Autodesk Inventor part; units mm, degrees
(part 2 of 2)
sketch "Sketch5" plane through (0, 0, 2) normal (0, 0, 1) x (1, 0, 0)
  line L0 (31.2247, -413) -> (28.338, -408) projected
  line L1 (28.338, -408) -> (31.2247, -403) projected
  line L2 (31.2247, -403) -> (36.9983, -403) projected
  line L3 (36.9983, -403) -> (39.885, -408) projected
  line L4 (39.885, -408) -> (36.9983, -413) projected
  line L5 (36.9983, -413) -> (31.2247, -413) projected
  line L6 (49.9886, -440.5) -> (52.8754, -445.5) projected
  line L7 (52.8754, -445.5) -> (49.9886, -450.5) projected
  line L8 (49.9886, -450.5) -> (44.2151, -450.5) projected
  line L9 (44.2151, -450.5) -> (41.3284, -445.5) projected
  line L10 (41.3284, -445.5) -> (44.2151, -440.5) projected
  line L11 (44.2151, -440.5) -> (49.9886, -440.5) projected
  line L12 (57.2247, -418) -> (62.9983, -418) projected
  line L13 (62.9983, -418) -> (65.885, -423) projected
  line L14 (65.885, -423) -> (62.9983, -428) projected
  line L15 (62.9983, -428) -> (57.2247, -428) projected
  line L16 (57.2247, -428) -> (54.338, -423) projected
  line L17 (54.338, -423) -> (57.2247, -418) projected
  line L18 (78.8754, -430.5) -> (75.9886, -435.5) projected
  line L19 (75.9886, -435.5) -> (70.2151, -435.5) projected
  line L20 (70.2151, -435.5) -> (67.3284, -430.5) projected
  line L21 (67.3284, -430.5) -> (70.2151, -425.5) projected
  line L22 (70.2151, -425.5) -> (75.9886, -425.5) projected
  line L23 (75.9886, -425.5) -> (78.8754, -430.5) projected
  line L24 (80.338, -438) -> (83.2247, -433) projected
  line L25 (83.2247, -433) -> (88.9983, -433) projected
  line L26 (88.9983, -433) -> (91.885, -438) projected
  line L27 (91.885, -438) -> (88.9983, -443) projected
  line L28 (88.9983, -443) -> (83.2247, -443) projected
  line L29 (83.2247, -443) -> (80.338, -438) projected
  line L30 (101.9886, -410.5) -> (104.8754, -415.5) projected
  line L31 (104.8754, -415.5) -> (101.9886, -420.5) projected
  line L32 (101.9886, -420.5) -> (96.2151, -420.5) projected
  line L33 (96.2151, -420.5) -> (93.3284, -415.5) projected
  line L34 (93.3284, -415.5) -> (96.2151, -410.5) projected
  line L35 (96.2151, -410.5) -> (101.9886, -410.5) projected
  line L36 (109.2247, -448) -> (114.9983, -448) projected
  line L37 (114.9983, -448) -> (117.885, -453) projected
  line L38 (117.885, -453) -> (114.9983, -458) projected
  line L39 (114.9983, -458) -> (109.2247, -458) projected
  line L40 (109.2247, -458) -> (106.338, -453) projected
  line L41 (106.338, -453) -> (109.2247, -448) projected
  line L42 (135.2247, -413) -> (132.338, -408) projected
  line L43 (132.338, -408) -> (135.2247, -403) projected
  line L44 (135.2247, -403) -> (140.9983, -403) projected
  line L45 (140.9983, -403) -> (143.885, -408) projected
  line L46 (143.885, -408) -> (140.9983, -413) projected
  line L47 (140.9983, -413) -> (135.2247, -413) projected
  line L48 (153.9886, -440.5) -> (156.8754, -445.5) projected
  line L49 (156.8754, -445.5) -> (153.9886, -450.5) projected
  line L50 (153.9886, -450.5) -> (148.2151, -450.5) projected
  line L51 (148.2151, -450.5) -> (145.3284, -445.5) projected
  line L52 (145.3284, -445.5) -> (148.2151, -440.5) projected
  line L53 (148.2151, -440.5) -> (153.9886, -440.5) projected
  line L54 (153.9886, -410.5) -> (156.8754, -415.5) projected
  line L55 (156.8754, -415.5) -> (153.9886, -420.5) projected
  line L56 (153.9886, -420.5) -> (148.2151, -420.5) projected
  line L57 (148.2151, -420.5) -> (145.3284, -415.5) projected
  line L58 (145.3284, -415.5) -> (148.2151, -410.5) projected
  line L59 (148.2151, -410.5) -> (153.9886, -410.5) projected
  line L60 (182.8754, -430.5) -> (179.9886, -435.5) projected
  line L61 (179.9886, -435.5) -> (174.2151, -435.5) projected
  line L62 (174.2151, -435.5) -> (171.3284, -430.5) projected
  line L63 (171.3284, -430.5) -> (174.2151, -425.5) projected
  line L64 (174.2151, -425.5) -> (179.9886, -425.5) projected
  line L65 (179.9886, -425.5) -> (182.8754, -430.5) projected
  line L66 (184.338, -438) -> (187.2247, -433) projected
  line L67 (187.2247, -433) -> (192.9983, -433) projected
  line L68 (192.9983, -433) -> (195.885, -438) projected
  line L69 (195.885, -438) -> (192.9983, -443) projected
  line L70 (192.9983, -443) -> (187.2247, -443) projected
  line L71 (187.2247, -443) -> (184.338, -438) projected
  line L72 (205.9886, -410.5) -> (208.8754, -415.5) projected
  line L73 (208.8754, -415.5) -> (205.9886, -420.5) projected
  line L74 (205.9886, -420.5) -> (200.2151, -420.5) projected
  line L75 (200.2151, -420.5) -> (197.3284, -415.5) projected
  line L76 (197.3284, -415.5) -> (200.2151, -410.5) projected
  line L77 (200.2151, -410.5) -> (205.9886, -410.5) projected
  line L78 (213.2247, -448) -> (218.9983, -448) projected
  line L79 (218.9983, -448) -> (221.885, -453) projected
  line L80 (221.885, -453) -> (218.9983, -458) projected
  line L81 (218.9983, -458) -> (213.2247, -458) projected
  line L82 (213.2247, -458) -> (210.338, -453) projected
  line L83 (210.338, -453) -> (213.2247, -448) projected
  line L84 (239.2247, -413) -> (236.338, -408) projected
  line L85 (236.338, -408) -> (239.2247, -403) projected
  line L86 (239.2247, -403) -> (244.9983, -403) projected
  line L87 (244.9983, -403) -> (247.885, -408) projected
  line L88 (247.885, -408) -> (244.9983, -413) projected
  line L89 (244.9983, -413) -> (239.2247, -413) projected
  line L90 (257.9886, -440.5) -> (260.8754, -445.5) projected
  line L91 (260.8754, -445.5) -> (257.9886, -450.5) projected
  line L92 (257.9886, -450.5) -> (252.2151, -450.5) projected
  line L93 (252.2151, -450.5) -> (249.3284, -445.5) projected
  line L94 (249.3284, -445.5) -> (252.2151, -440.5) projected
  line L95 (252.2151, -440.5) -> (257.9886, -440.5) projected
  line L96 (265.2247, -418) -> (270.9983, -418) projected
  line L97 (270.9983, -418) -> (273.885, -423) projected
  line L98 (273.885, -423) -> (270.9983, -428) projected
  line L99 (270.9983, -428) -> (265.2247, -428) projected
  line L100 (265.2247, -428) -> (262.338, -423) projected
  line L101 (262.338, -423) -> (265.2247, -418) projected
  line L102 (291.2247, -448) -> (296.9983, -448) projected
  line L103 (296.9983, -448) -> (299.885, -453) projected
  line L104 (299.885, -453) -> (296.9983, -458) projected
  line L105 (296.9983, -458) -> (291.2247, -458) projected
  line L106 (291.2247, -458) -> (288.338, -453) projected
  line L107 (288.338, -453) -> (291.2247, -448) projected
  line L108 (343.2247, -448) -> (348.9983, -448) projected
  line L109 (348.9983, -448) -> (351.885, -453) projected
  line L110 (351.885, -453) -> (348.9983, -458) projected
  line L111 (348.9983, -458) -> (343.2247, -458) projected
  line L112 (343.2247, -458) -> (340.338, -453) projected
  line L113 (340.338, -453) -> (343.2247, -448) projected
  line L114 (335.9886, -410.5) -> (338.8754, -415.5) projected
  line L115 (338.8754, -415.5) -> (335.9886, -420.5) projected
  line L116 (335.9886, -420.5) -> (330.2151, -420.5) projected
  line L117 (330.2151, -420.5) -> (327.3284, -415.5) projected
  line L118 (327.3284, -415.5) -> (330.2151, -410.5) projected
  line L119 (330.2151, -410.5) -> (335.9886, -410.5) projected
  line L120 (286.8754, -430.5) -> (283.9886, -435.5) projected
  line L121 (283.9886, -435.5) -> (278.2151, -435.5) projected
  line L122 (278.2151, -435.5) -> (275.3284, -430.5) projected
  line L123 (275.3284, -430.5) -> (278.2151, -425.5) projected
  line L124 (278.2151, -425.5) -> (283.9886, -425.5) projected
  line L125 (283.9886, -425.5) -> (286.8754, -430.5) projected
  line L126 (309.9886, -410.5) -> (312.8754, -415.5) projected
  line L127 (312.8754, -415.5) -> (309.9886, -420.5) projected
  line L128 (309.9886, -420.5) -> (304.2151, -420.5) projected
  line L129 (304.2151, -420.5) -> (301.3284, -415.5) projected
  line L130 (301.3284, -415.5) -> (304.2151, -410.5) projected
  line L131 (304.2151, -410.5) -> (309.9886, -410.5) projected
  line L132 (5.2247, -433) -> (10.9983, -433) projected
  line L133 (10.9983, -433) -> (13.885, -438) projected
  line L134 (13.885, -438) -> (10.9983, -443) projected
  line L135 (10.9983, -443) -> (5.2247, -443) projected
  line L136 (5.2247, -443) -> (2.338, -438) projected
  line L137 (2.338, -438) -> (5.2247, -433) projected
  line L138 (23.9886, -440.5) -> (26.8754, -445.5) projected
  line L139 (26.8754, -445.5) -> (23.9886, -450.5) projected
  line L140 (23.9886, -450.5) -> (18.2151, -450.5) projected
  line L141 (18.2151, -450.5) -> (15.3284, -445.5) projected
  line L142 (15.3284, -445.5) -> (18.2151, -440.5) projected
  line L143 (18.2151, -440.5) -> (23.9886, -440.5) projected
  line L144 (10.9983, -428) -> (5.2247, -428) projected
  line L145 (5.2247, -428) -> (2.338, -423) projected
  line L146 (2.338, -423) -> (5.2247, -418) projected
  line L147 (5.2247, -418) -> (10.9983, -418) projected
  line L148 (10.9983, -418) -> (13.885, -423) projected
  line L149 (13.885, -423) -> (10.9983, -428) projected
  line L150 (317.2247, -418) -> (322.9983, -418) projected
  line L151 (322.9983, -418) -> (325.885, -423) projected
  line L152 (325.885, -423) -> (322.9983, -428) projected
  line L153 (322.9983, -428) -> (317.2247, -428) projected
  line L154 (317.2247, -428) -> (314.338, -423) projected
  line L155 (314.338, -423) -> (317.2247, -418) projected
  line L156 (291.2247, -418) -> (296.9983, -418) projected
  line L157 (296.9983, -418) -> (299.885, -423) projected
  line L158 (299.885, -423) -> (296.9983, -428) projected
  line L159 (296.9983, -428) -> (291.2247, -428) projected
  line L160 (291.2247, -428) -> (288.338, -423) projected
  line L161 (288.338, -423) -> (291.2247, -418) projected
  line L162 (317.2247, -413) -> (314.338, -408) projected
  line L163 (314.338, -408) -> (317.2247, -403) projected
  line L164 (317.2247, -403) -> (322.9983, -403) projected
  line L165 (322.9983, -403) -> (325.885, -408) projected
  line L166 (325.885, -408) -> (322.9983, -413) projected
  line L167 (322.9983, -413) -> (317.2247, -413) projected
  line L168 (340.338, -438) -> (343.2247, -433) projected
  line L169 (343.2247, -433) -> (348.9983, -433) projected
  line L170 (348.9983, -433) -> (351.885, -438) projected
  line L171 (351.885, -438) -> (348.9983, -443) projected
  line L172 (348.9983, -443) -> (343.2247, -443) projected
  line L173 (343.2247, -443) -> (340.338, -438) projected
  line L174 (309.9886, -440.5) -> (312.8754, -445.5) projected
  line L175 (312.8754, -445.5) -> (309.9886, -450.5) projected
  line L176 (309.9886, -450.5) -> (304.2151, -450.5) projected
  line L177 (304.2151, -450.5) -> (301.3284, -445.5) projected
  line L178 (301.3284, -445.5) -> (304.2151, -440.5) projected
  line L179 (304.2151, -440.5) -> (309.9886, -440.5) projected
  line L180 (262.338, -438) -> (265.2247, -433) projected
  line L181 (265.2247, -433) -> (270.9983, -433) projected
  line L182 (270.9983, -433) -> (273.885, -438) projected
  line L183 (273.885, -438) -> (270.9983, -443) projected
  line L184 (270.9983, -443) -> (265.2247, -443) projected
  line L185 (265.2247, -443) -> (262.338, -438) projected
  line L186 (260.8754, -430.5) -> (257.9886, -435.5) projected
  line L187 (257.9886, -435.5) -> (252.2151, -435.5) projected
  line L188 (252.2151, -435.5) -> (249.3284, -430.5) projected
  line L189 (249.3284, -430.5) -> (252.2151, -425.5) projected
  line L190 (252.2151, -425.5) -> (257.9886, -425.5) projected
  line L191 (257.9886, -425.5) -> (260.8754, -430.5) projected
  line L192 (239.2247, -418) -> (244.9983, -418) projected
  line L193 (244.9983, -418) -> (247.885, -423) projected
  line L194 (247.885, -423) -> (244.9983, -428) projected
  line L195 (244.9983, -428) -> (239.2247, -428) projected
  line L196 (239.2247, -428) -> (236.338, -423) projected
  line L197 (236.338, -423) -> (239.2247, -418) projected
  line L198 (231.9886, -440.5) -> (234.8754, -445.5) projected
  line L199 (234.8754, -445.5) -> (231.9886, -450.5) projected
  line L200 (231.9886, -450.5) -> (226.2151, -450.5) projected
  line L201 (226.2151, -450.5) -> (223.3284, -445.5) projected
  line L202 (223.3284, -445.5) -> (226.2151, -440.5) projected
  line L203 (226.2151, -440.5) -> (231.9886, -440.5) projected
  line L204 (213.2247, -413) -> (210.338, -408) projected
  line L205 (210.338, -408) -> (213.2247, -403) projected
  line L206 (213.2247, -403) -> (218.9983, -403) projected
  line L207 (218.9983, -403) -> (221.885, -408) projected
  line L208 (221.885, -408) -> (218.9983, -413) projected
  line L209 (218.9983, -413) -> (213.2247, -413) projected
  line L210 (187.2247, -448) -> (192.9983, -448) projected
  line L211 (192.9983, -448) -> (195.885, -453) projected
  line L212 (195.885, -453) -> (192.9983, -458) projected
  line L213 (192.9983, -458) -> (187.2247, -458) projected
  line L214 (187.2247, -458) -> (184.338, -453) projected
  line L215 (184.338, -453) -> (187.2247, -448) projected
  line L216 (179.9886, -410.5) -> (182.8754, -415.5) projected
  line L217 (182.8754, -415.5) -> (179.9886, -420.5) projected
  line L218 (179.9886, -420.5) -> (174.2151, -420.5) projected
  line L219 (174.2151, -420.5) -> (171.3284, -415.5) projected
  line L220 (171.3284, -415.5) -> (174.2151, -410.5) projected
  line L221 (174.2151, -410.5) -> (179.9886, -410.5) projected
  line L222 (161.2247, -413) -> (158.338, -408) projected
  line L223 (158.338, -408) -> (161.2247, -403) projected
  line L224 (161.2247, -403) -> (166.9983, -403) projected
  line L225 (166.9983, -403) -> (169.885, -408) projected
  line L226 (169.885, -408) -> (166.9983, -413) projected
  line L227 (166.9983, -413) -> (161.2247, -413) projected
  line L228 (161.2247, -448) -> (166.9983, -448) projected
  line L229 (166.9983, -448) -> (169.885, -453) projected
  line L230 (169.885, -453) -> (166.9983, -458) projected
  line L231 (166.9983, -458) -> (161.2247, -458) projected
  line L232 (161.2247, -458) -> (158.338, -453) projected
  line L233 (158.338, -453) -> (161.2247, -448) projected
  line L234 (135.2247, -418) -> (140.9983, -418) projected
  line L235 (140.9983, -418) -> (143.885, -423) projected
  line L236 (143.885, -423) -> (140.9983, -428) projected
  line L237 (140.9983, -428) -> (135.2247, -428) projected
  line L238 (135.2247, -428) -> (132.338, -423) projected
  line L239 (132.338, -423) -> (135.2247, -418) projected
  line L240 (127.9886, -440.5) -> (130.8754, -445.5) projected
  line L241 (130.8754, -445.5) -> (127.9886, -450.5) projected
  line L242 (127.9886, -450.5) -> (122.2151, -450.5) projected
  line L243 (122.2151, -450.5) -> (119.3284, -445.5) projected
  line L244 (119.3284, -445.5) -> (122.2151, -440.5) projected
  line L245 (122.2151, -440.5) -> (127.9886, -440.5) projected
  line L246 (109.2247, -413) -> (106.338, -408) projected
  line L247 (106.338, -408) -> (109.2247, -403) projected
  line L248 (109.2247, -403) -> (114.9983, -403) projected
  line L249 (114.9983, -403) -> (117.885, -408) projected
  line L250 (117.885, -408) -> (114.9983, -413) projected
  line L251 (114.9983, -413) -> (109.2247, -413) projected
  line L252 (83.2247, -448) -> (88.9983, -448) projected
  line L253 (88.9983, -448) -> (91.885, -453) projected
  line L254 (91.885, -453) -> (88.9983, -458) projected
  line L255 (88.9983, -458) -> (83.2247, -458) projected
  line L256 (83.2247, -458) -> (80.338, -453) projected
  line L257 (80.338, -453) -> (83.2247, -448) projected
  line L258 (75.9886, -410.5) -> (78.8754, -415.5) projected
  line L259 (78.8754, -415.5) -> (75.9886, -420.5) projected
  line L260 (75.9886, -420.5) -> (70.2151, -420.5) projected
  line L261 (70.2151, -420.5) -> (67.3284, -415.5) projected
  line L262 (67.3284, -415.5) -> (70.2151, -410.5) projected
  line L263 (70.2151, -410.5) -> (75.9886, -410.5) projected
  line L264 (54.338, -438) -> (57.2247, -433) projected
  line L265 (57.2247, -433) -> (62.9983, -433) projected
  line L266 (62.9983, -433) -> (65.885, -438) projected
  line L267 (65.885, -438) -> (62.9983, -443) projected
  line L268 (62.9983, -443) -> (57.2247, -443) projected
  line L269 (57.2247, -443) -> (54.338, -438) projected
  line L270 (52.8754, -430.5) -> (49.9886, -435.5) projected
  line L271 (49.9886, -435.5) -> (44.2151, -435.5) projected
  line L272 (44.2151, -435.5) -> (41.3284, -430.5) projected
  line L273 (41.3284, -430.5) -> (44.2151, -425.5) projected
  line L274 (44.2151, -425.5) -> (49.9886, -425.5) projected
  line L275 (49.9886, -425.5) -> (52.8754, -430.5) projected
  line L276 (31.2247, -418) -> (36.9983, -418) projected
  line L277 (36.9983, -418) -> (39.885, -423) projected
  line L278 (39.885, -423) -> (36.9983, -428) projected
  line L279 (36.9983, -428) -> (31.2247, -428) projected
  line L280 (31.2247, -428) -> (28.338, -423) projected
  line L281 (28.338, -423) -> (31.2247, -418) projected
  line L282 (23.9886, -420.5) -> (18.2151, -420.5) projected
  line L283 (18.2151, -420.5) -> (15.3284, -415.5) projected
  line L284 (15.3284, -415.5) -> (18.2151, -410.5) projected
  line L285 (18.2151, -410.5) -> (23.9886, -410.5) projected
  line L286 (23.9886, -410.5) -> (26.8754, -415.5) projected
  line L287 (26.8754, -415.5) -> (23.9886, -420.5) projected
  line L288 (31.2247, -448) -> (36.9983, -448) projected
  line L289 (36.9983, -448) -> (39.885, -453) projected
  line L290 (39.885, -453) -> (36.9983, -458) projected
  line L291 (36.9983, -458) -> (31.2247, -458) projected
  line L292 (31.2247, -458) -> (28.338, -453) projected
  line L293 (28.338, -453) -> (31.2247, -448) projected
  line L294 (57.2247, -413) -> (54.338, -408) projected
  line L295 (54.338, -408) -> (57.2247, -403) projected
  line L296 (57.2247, -403) -> (62.9983, -403) projected
  line L297 (62.9983, -403) -> (65.885, -408) projected
  line L298 (65.885, -408) -> (62.9983, -413) projected
  line L299 (62.9983, -413) -> (57.2247, -413) projected
  line L300 (75.9886, -440.5) -> (78.8754, -445.5) projected
  line L301 (78.8754, -445.5) -> (75.9886, -450.5) projected
  line L302 (75.9886, -450.5) -> (70.2151, -450.5) projected
  line L303 (70.2151, -450.5) -> (67.3284, -445.5) projected
  line L304 (67.3284, -445.5) -> (70.2151, -440.5) projected
  line L305 (70.2151, -440.5) -> (75.9886, -440.5) projected
  line L306 (83.2247, -418) -> (88.9983, -418) projected
  line L307 (88.9983, -418) -> (91.885, -423) projected
  line L308 (91.885, -423) -> (88.9983, -428) projected
  line L309 (88.9983, -428) -> (83.2247, -428) projected
  line L310 (83.2247, -428) -> (80.338, -423) projected
  line L311 (80.338, -423) -> (83.2247, -418) projected
  line L312 (104.8754, -430.5) -> (101.9886, -435.5) projected
  line L313 (101.9886, -435.5) -> (96.2151, -435.5) projected
  line L314 (96.2151, -435.5) -> (93.3284, -430.5) projected
  line L315 (93.3284, -430.5) -> (96.2151, -425.5) projected
  line L316 (96.2151, -425.5) -> (101.9886, -425.5) projected
  line L317 (101.9886, -425.5) -> (104.8754, -430.5) projected
  line L318 (106.338, -438) -> (109.2247, -433) projected
  line L319 (109.2247, -433) -> (114.9983, -433) projected
  line L320 (114.9983, -433) -> (117.885, -438) projected
  line L321 (117.885, -438) -> (114.9983, -443) projected
  line L322 (114.9983, -443) -> (109.2247, -443) projected
  line L323 (109.2247, -443) -> (106.338, -438) projected
  line L324 (127.9886, -410.5) -> (130.8754, -415.5) projected
  line L325 (130.8754, -415.5) -> (127.9886, -420.5) projected
  line L326 (127.9886, -420.5) -> (122.2151, -420.5) projected
  line L327 (122.2151, -420.5) -> (119.3284, -415.5) projected
  line L328 (119.3284, -415.5) -> (122.2151, -410.5) projected
  line L329 (122.2151, -410.5) -> (127.9886, -410.5) projected
  line L330 (135.2247, -448) -> (140.9983, -448) projected
  line L331 (140.9983, -448) -> (143.885, -453) projected
  line L332 (143.885, -453) -> (140.9983, -458) projected
  line L333 (140.9983, -458) -> (135.2247, -458) projected
  line L334 (135.2247, -458) -> (132.338, -453) projected
  line L335 (132.338, -453) -> (135.2247, -448) projected
  line L336 (156.8754, -430.5) -> (153.9886, -435.5) projected
  line L337 (153.9886, -435.5) -> (148.2151, -435.5) projected
  line L338 (148.2151, -435.5) -> (145.3284, -430.5) projected
  line L339 (145.3284, -430.5) -> (148.2151, -425.5) projected
  line L340 (148.2151, -425.5) -> (153.9886, -425.5) projected
  line L341 (153.9886, -425.5) -> (156.8754, -430.5) projected
  line L342 (179.9886, -440.5) -> (182.8754, -445.5) projected
  line L343 (182.8754, -445.5) -> (179.9886, -450.5) projected
  line L344 (179.9886, -450.5) -> (174.2151, -450.5) projected
  line L345 (174.2151, -450.5) -> (171.3284, -445.5) projected
  line L346 (171.3284, -445.5) -> (174.2151, -440.5) projected
  line L347 (174.2151, -440.5) -> (179.9886, -440.5) projected
  line L348 (187.2247, -418) -> (192.9983, -418) projected
  line L349 (192.9983, -418) -> (195.885, -423) projected
  line L350 (195.885, -423) -> (192.9983, -428) projected
  line L351 (192.9983, -428) -> (187.2247, -428) projected
  line L352 (187.2247, -428) -> (184.338, -423) projected
  line L353 (184.338, -423) -> (187.2247, -418) projected
  line L354 (208.8754, -430.5) -> (205.9886, -435.5) projected
  line L355 (205.9886, -435.5) -> (200.2151, -435.5) projected
  line L356 (200.2151, -435.5) -> (197.3284, -430.5) projected
  line L357 (197.3284, -430.5) -> (200.2151, -425.5) projected
  line L358 (200.2151, -425.5) -> (205.9886, -425.5) projected
  line L359 (205.9886, -425.5) -> (208.8754, -430.5) projected
  line L360 (210.338, -438) -> (213.2247, -433) projected
  line L361 (213.2247, -433) -> (218.9983, -433) projected
  line L362 (218.9983, -433) -> (221.885, -438) projected
  line L363 (221.885, -438) -> (218.9983, -443) projected
  line L364 (218.9983, -443) -> (213.2247, -443) projected
  line L365 (213.2247, -443) -> (210.338, -438) projected
  line L366 (231.9886, -410.5) -> (234.8754, -415.5) projected
  line L367 (234.8754, -415.5) -> (231.9886, -420.5) projected
  line L368 (231.9886, -420.5) -> (226.2151, -420.5) projected
  line L369 (226.2151, -420.5) -> (223.3284, -415.5) projected
  line L370 (223.3284, -415.5) -> (226.2151, -410.5) projected
  line L371 (226.2151, -410.5) -> (231.9886, -410.5) projected
  line L372 (239.2247, -448) -> (244.9983, -448) projected
  line L373 (244.9983, -448) -> (247.885, -453) projected
  line L374 (247.885, -453) -> (244.9983, -458) projected
  line L375 (244.9983, -458) -> (239.2247, -458) projected
  line L376 (239.2247, -458) -> (236.338, -453) projected
  line L377 (236.338, -453) -> (239.2247, -448) projected
  line L378 (265.2247, -413) -> (262.338, -408) projected
  line L379 (262.338, -408) -> (265.2247, -403) projected
  line L380 (265.2247, -403) -> (270.9983, -403) projected
  line L381 (270.9983, -403) -> (273.885, -408) projected
  line L382 (273.885, -408) -> (270.9983, -413) projected
  line L383 (270.9983, -413) -> (265.2247, -413) projected
  line L384 (283.9886, -440.5) -> (286.8754, -445.5) projected
  line L385 (286.8754, -445.5) -> (283.9886, -450.5) projected
  line L386 (283.9886, -450.5) -> (278.2151, -450.5) projected
  line L387 (278.2151, -450.5) -> (275.3284, -445.5) projected
  line L388 (275.3284, -445.5) -> (278.2151, -440.5) projected
  line L389 (278.2151, -440.5) -> (283.9886, -440.5) projected
  line L390 (335.9886, -440.5) -> (338.8754, -445.5) projected
  line L391 (338.8754, -445.5) -> (335.9886, -450.5) projected
  line L392 (335.9886, -450.5) -> (330.2151, -450.5) projected
  line L393 (330.2151, -450.5) -> (327.3284, -445.5) projected
  line L394 (327.3284, -445.5) -> (330.2151, -440.5) projected
  line L395 (330.2151, -440.5) -> (335.9886, -440.5) projected
  line L396 (343.2247, -413) -> (340.338, -408) projected
  line L397 (340.338, -408) -> (343.2247, -403) projected
  line L398 (343.2247, -403) -> (348.9983, -403) projected
  line L399 (348.9983, -403) -> (351.885, -408) projected
  line L400 (351.885, -408) -> (348.9983, -413) projected
  line L401 (348.9983, -413) -> (343.2247, -413) projected
  line L402 (283.9886, -410.5) -> (286.8754, -415.5) projected
  line L403 (286.8754, -415.5) -> (283.9886, -420.5) projected
  line L404 (283.9886, -420.5) -> (278.2151, -420.5) projected
  line L405 (278.2151, -420.5) -> (275.3284, -415.5) projected
  line L406 (275.3284, -415.5) -> (278.2151, -410.5) projected
  line L407 (278.2151, -410.5) -> (283.9886, -410.5) projected
  line L408 (312.8754, -430.5) -> (309.9886, -435.5) projected
  line L409 (309.9886, -435.5) -> (304.2151, -435.5) projected
  line L410 (304.2151, -435.5) -> (301.3284, -430.5) projected
  line L411 (301.3284, -430.5) -> (304.2151, -425.5) projected
  line L412 (304.2151, -425.5) -> (309.9886, -425.5) projected
  line L413 (309.9886, -425.5) -> (312.8754, -430.5) projected
  line L414 (338.8754, -430.5) -> (335.9886, -435.5) projected
  line L415 (335.9886, -435.5) -> (330.2151, -435.5) projected
  line L416 (330.2151, -435.5) -> (327.3284, -430.5) projected
  line L417 (327.3284, -430.5) -> (330.2151, -425.5) projected
  line L418 (330.2151, -425.5) -> (335.9886, -425.5) projected
  line L419 (335.9886, -425.5) -> (338.8754, -430.5) projected
  line L420 (23.9886, -435.5) -> (18.2151, -435.5) projected
  line L421 (18.2151, -435.5) -> (15.3284, -430.5) projected
  line L422 (15.3284, -430.5) -> (18.2151, -425.5) projected
  line L423 (18.2151, -425.5) -> (23.9886, -425.5) projected
  line L424 (23.9886, -425.5) -> (26.8754, -430.5) projected
  line L425 (26.8754, -430.5) -> (23.9886, -435.5) projected
  line L426 (5.2247, -448) -> (10.9983, -448) projected
  line L427 (10.9983, -448) -> (13.885, -453) projected
  line L428 (13.885, -453) -> (10.9983, -458) projected
  line L429 (10.9983, -458) -> (5.2247, -458) projected
  line L430 (5.2247, -458) -> (2.338, -453) projected
  line L431 (2.338, -453) -> (5.2247, -448) projected
  line L432 (314.338, -438) -> (317.2247, -433) projected
  line L433 (317.2247, -433) -> (322.9983, -433) projected
  line L434 (322.9983, -433) -> (325.885, -438) projected
  line L435 (325.885, -438) -> (322.9983, -443) projected
  line L436 (322.9983, -443) -> (317.2247, -443) projected
  line L437 (317.2247, -443) -> (314.338, -438) projected
  line L438 (288.338, -438) -> (291.2247, -433) projected
  line L439 (291.2247, -433) -> (296.9983, -433) projected
  line L440 (296.9983, -433) -> (299.885, -438) projected
  line L441 (299.885, -438) -> (296.9983, -443) projected
  line L442 (296.9983, -443) -> (291.2247, -443) projected
  line L443 (291.2247, -443) -> (288.338, -438) projected
  line L444 (291.2247, -413) -> (288.338, -408) projected
  line L445 (288.338, -408) -> (291.2247, -403) projected
  line L446 (291.2247, -403) -> (296.9983, -403) projected
  line L447 (296.9983, -403) -> (299.885, -408) projected
  line L448 (299.885, -408) -> (296.9983, -413) projected
  line L449 (296.9983, -413) -> (291.2247, -413) projected
  line L450 (343.2247, -418) -> (348.9983, -418) projected
  line L451 (348.9983, -418) -> (351.885, -423) projected
  line L452 (351.885, -423) -> (348.9983, -428) projected
  line L453 (348.9983, -428) -> (343.2247, -428) projected
  line L454 (343.2247, -428) -> (340.338, -423) projected
  line L455 (340.338, -423) -> (343.2247, -418) projected
  line L456 (317.2247, -448) -> (322.9983, -448) projected
  line L457 (322.9983, -448) -> (325.885, -453) projected
  line L458 (325.885, -453) -> (322.9983, -458) projected
  line L459 (322.9983, -458) -> (317.2247, -458) projected
  line L460 (317.2247, -458) -> (314.338, -453) projected
  line L461 (314.338, -453) -> (317.2247, -448) projected
  line L462 (265.2247, -448) -> (270.9983, -448) projected
  line L463 (270.9983, -448) -> (273.885, -453) projected
  line L464 (273.885, -453) -> (270.9983, -458) projected
  line L465 (270.9983, -458) -> (265.2247, -458) projected
  line L466 (265.2247, -458) -> (262.338, -453) projected
  line L467 (262.338, -453) -> (265.2247, -448) projected
  line L468 (257.9886, -410.5) -> (260.8754, -415.5) projected
  line L469 (260.8754, -415.5) -> (257.9886, -420.5) projected
  line L470 (257.9886, -420.5) -> (252.2151, -420.5) projected
  line L471 (252.2151, -420.5) -> (249.3284, -415.5) projected
  line L472 (249.3284, -415.5) -> (252.2151, -410.5) projected
  line L473 (252.2151, -410.5) -> (257.9886, -410.5) projected
  line L474 (236.338, -438) -> (239.2247, -433) projected
  line L475 (239.2247, -433) -> (244.9983, -433) projected
  line L476 (244.9983, -433) -> (247.885, -438) projected
  line L477 (247.885, -438) -> (244.9983, -443) projected
  line L478 (244.9983, -443) -> (239.2247, -443) projected
  line L479 (239.2247, -443) -> (236.338, -438) projected
  line L480 (234.8754, -430.5) -> (231.9886, -435.5) projected
  line L481 (231.9886, -435.5) -> (226.2151, -435.5) projected
  line L482 (226.2151, -435.5) -> (223.3284, -430.5) projected
  line L483 (223.3284, -430.5) -> (226.2151, -425.5) projected
  line L484 (226.2151, -425.5) -> (231.9886, -425.5) projected
  line L485 (231.9886, -425.5) -> (234.8754, -430.5) projected
  line L486 (213.2247, -418) -> (218.9983, -418) projected
  line L487 (218.9983, -418) -> (221.885, -423) projected
  line L488 (221.885, -423) -> (218.9983, -428) projected
  line L489 (218.9983, -428) -> (213.2247, -428) projected
  line L490 (213.2247, -428) -> (210.338, -423) projected
  line L491 (210.338, -423) -> (213.2247, -418) projected
  line L492 (205.9886, -440.5) -> (208.8754, -445.5) projected
  line L493 (208.8754, -445.5) -> (205.9886, -450.5) projected
  line L494 (205.9886, -450.5) -> (200.2151, -450.5) projected
  line L495 (200.2151, -450.5) -> (197.3284, -445.5) projected
  line L496 (197.3284, -445.5) -> (200.2151, -440.5) projected
  line L497 (200.2151, -440.5) -> (205.9886, -440.5) projected
  line L498 (187.2247, -413) -> (184.338, -408) projected
  line L499 (184.338, -408) -> (187.2247, -403) projected
  line L500 (187.2247, -403) -> (192.9983, -403) projected
  line L501 (192.9983, -403) -> (195.885, -408) projected
  line L502 (195.885, -408) -> (192.9983, -413) projected
  line L503 (192.9983, -413) -> (187.2247, -413) projected
  line L504 (161.2247, -418) -> (166.9983, -418) projected
  line L505 (166.9983, -418) -> (169.885, -423) projected
  line L506 (169.885, -423) -> (166.9983, -428) projected
  line L507 (166.9983, -428) -> (161.2247, -428) projected
  line L508 (161.2247, -428) -> (158.338, -423) projected
  line L509 (158.338, -423) -> (161.2247, -418) projected
  line L510 (158.338, -438) -> (161.2247, -433) projected
  line L511 (161.2247, -433) -> (166.9983, -433) projected
  line L512 (166.9983, -433) -> (169.885, -438) projected
  line L513 (169.885, -438) -> (166.9983, -443) projected
  line L514 (166.9983, -443) -> (161.2247, -443) projected
  line L515 (161.2247, -443) -> (158.338, -438) projected
  line L516 (132.338, -438) -> (135.2247, -433) projected
  line L517 (135.2247, -433) -> (140.9983, -433) projected
  line L518 (140.9983, -433) -> (143.885, -438) projected
  line L519 (143.885, -438) -> (140.9983, -443) projected
  line L520 (140.9983, -443) -> (135.2247, -443) projected
  line L521 (135.2247, -443) -> (132.338, -438) projected
  line L522 (130.8754, -430.5) -> (127.9886, -435.5) projected
  line L523 (127.9886, -435.5) -> (122.2151, -435.5) projected
  line L524 (122.2151, -435.5) -> (119.3284, -430.5) projected
  line L525 (119.3284, -430.5) -> (122.2151, -425.5) projected
  line L526 (122.2151, -425.5) -> (127.9886, -425.5) projected
  line L527 (127.9886, -425.5) -> (130.8754, -430.5) projected
  line L528 (109.2247, -418) -> (114.9983, -418) projected
  line L529 (114.9983, -418) -> (117.885, -423) projected
  line L530 (117.885, -423) -> (114.9983, -428) projected
  line L531 (114.9983, -428) -> (109.2247, -428) projected
  line L532 (109.2247, -428) -> (106.338, -423) projected
  line L533 (106.338, -423) -> (109.2247, -418) projected
  line L534 (101.9886, -440.5) -> (104.8754, -445.5) projected
  line L535 (104.8754, -445.5) -> (101.9886, -450.5) projected
  line L536 (101.9886, -450.5) -> (96.2151, -450.5) projected
  line L537 (96.2151, -450.5) -> (93.3284, -445.5) projected
  line L538 (93.3284, -445.5) -> (96.2151, -440.5) projected
  line L539 (96.2151, -440.5) -> (101.9886, -440.5) projected
  line L540 (83.2247, -413) -> (80.338, -408) projected
  line L541 (80.338, -408) -> (83.2247, -403) projected
  line L542 (83.2247, -403) -> (88.9983, -403) projected
  line L543 (88.9983, -403) -> (91.885, -408) projected
  line L544 (91.885, -408) -> (88.9983, -413) projected
  line L545 (88.9983, -413) -> (83.2247, -413) projected
  line L546 (57.2247, -448) -> (62.9983, -448) projected
  line L547 (62.9983, -448) -> (65.885, -453) projected
  line L548 (65.885, -453) -> (62.9983, -458) projected
  line L549 (62.9983, -458) -> (57.2247, -458) projected
  line L550 (57.2247, -458) -> (54.338, -453) projected
  line L551 (54.338, -453) -> (57.2247, -448) projected
  line L552 (49.9886, -410.5) -> (52.8754, -415.5) projected
  line L553 (52.8754, -415.5) -> (49.9886, -420.5) projected
  line L554 (49.9886, -420.5) -> (44.2151, -420.5) projected
  line L555 (44.2151, -420.5) -> (41.3284, -415.5) projected
  line L556 (41.3284, -415.5) -> (44.2151, -410.5) projected
  line L557 (44.2151, -410.5) -> (49.9886, -410.5) projected
  line L558 (28.338, -438) -> (31.2247, -433) projected
  line L559 (31.2247, -433) -> (36.9983, -433) projected
  line L560 (36.9983, -433) -> (39.885, -438) projected
  line L561 (39.885, -438) -> (36.9983, -443) projected
  line L562 (36.9983, -443) -> (31.2247, -443) projected
  line L563 (31.2247, -443) -> (28.338, -438) projected
  line L564 (10.9983, -413) -> (5.2247, -413) projected
  line L565 (5.2247, -413) -> (2.338, -408) projected
  line L566 (2.338, -408) -> (5.2247, -403) projected
  line L567 (5.2247, -403) -> (10.9983, -403) projected
  line L568 (10.9983, -403) -> (13.885, -408) projected
  line L569 (13.885, -408) -> (10.9983, -413) projected
  circle A0 centre (260, -90.5) radius 15 projected
  circle A1 centre (180, -90.5) radius 15 projected
  circle A2 centre (100, -90.5) radius 15 projected
  circle A3 centre (84.5, -106) radius 1.75 projected
  circle A4 centre (115.5, -75) radius 1.75 projected
  circle A5 centre (164.5, -106) radius 1.75 projected
  circle A6 centre (195.5, -75) radius 1.75 projected
  circle A7 centre (275.5, -106) radius 1.75 projected
  circle A8 centre (275.5, -75) radius 1.75 projected
  circle A9 centre (244.5, -75) radius 1.75 projected
  circle A10 centre (244.5, -106) radius 1.75 projected
  circle A11 centre (164.5, -75) radius 1.75 projected
  circle A12 centre (195.5, -106) radius 1.75 projected
  circle A13 centre (84.5, -75) radius 1.75 projected
  circle A14 centre (115.5, -106) radius 1.75 projected
  line L570 (375, -480) -> (375, 0) projected
  line L571 (375, 0) -> (-15, 0) projected
  line L572 (-15, 0) -> (-15, -480) projected
  line L573 (-15, -480) -> (375, -480) projected
  circle A15 centre (100, -25) radius 1.75 projected
  circle A16 centre (180, -7.5) radius 1.75 projected
  circle A17 centre (-7.5, -65) radius 1.75 projected
  circle A18 centre (-7.5, -415) radius 1.75 projected
  circle A19 centre (367.5, -65) radius 1.75 projected
  circle A20 centre (367.5, -415) radius 1.75 projected
  circle A21 centre (50, -7.5) radius 1.75 projected
  circle A22 centre (310, -7.5) radius 1.75 projected
  circle A23 centre (310, -472.5) radius 1.75 projected
  circle A24 centre (50, -472.5) radius 1.75 projected
  circle A25 centre (180, -25) radius 1.75 projected
  circle A26 centre (260, -25) radius 1.75 projected
  line L574 (-15, -280) -> (375, -280) construction
  line L575 (375, -280) -> (375, -330) construction
  line L576 (375, -330) -> (-15, -330) construction
  line L577 (-15, -330) -> (-15, -280) construction
  line L578 (46.6125, -329.9768) -> (40.3392, -323.7035)
  line L579 (40.3392, -323.7035) -> (40.3392, -279.9768)
  line L580 (40.3392, -279.9768) -> (56.789, -279.9768)
  line L581 (56.789, -279.9768) -> (56.789, -329.9768)
  line L582 (56.789, -329.9768) -> (46.6125, -329.9768)
  line L583 (60.3206, -329.9768) -> (60.3206, -316.1756)
  line L584 (60.3206, -316.1756) -> (92.5697, -316.1756)
  line L585 (92.5697, -316.1756) -> (92.5697, -329.9768)
  line L586 (92.5697, -329.9768) -> (60.3206, -329.9768)
  line L587 (129.3262, -329.9303) -> (104.7444, -329.9303)
  line L588 (104.7444, -329.9303) -> (96.8913, -322.0771)
  line L589 (96.8913, -322.0771) -> (96.8913, -294.289)
  line L590 (96.8913, -294.289) -> (113.5734, -294.289)
  line L591 (113.5734, -294.289) -> (113.5734, -316.1292)
  line L592 (113.5734, -316.1292) -> (129.3262, -316.1292)
  line L593 (129.3262, -316.1292) -> (129.3262, -329.9303)
  line L594 (149.447, -329.9303) -> (132.7649, -329.9303)
  line L595 (132.7649, -329.9303) -> (132.7649, -294.289)
  line L596 (132.7649, -294.289) -> (149.447, -294.289)
  line L597 (149.447, -294.289) -> (149.447, -329.9303)
  line L598 (170.3113, -329.9768) -> (159.9954, -329.9768)
  line L599 (159.9954, -329.9768) -> (153.7221, -323.7035)
  line L600 (153.7221, -323.7035) -> (153.7221, -286.25)
  line L601 (153.7221, -286.25) -> (159.9954, -279.9768)
  line L602 (159.9954, -279.9768) -> (170.3113, -279.9768)
  line L603 (170.3113, -279.9768) -> (170.3113, -329.9768)
  line L604 (206.2779, -294.4284) -> (173.8429, -294.4284)
  line L605 (173.8429, -294.4284) -> (173.8429, -279.9768)
  line L606 (173.8429, -279.9768) -> (206.2779, -279.9768)
  line L607 (206.2779, -279.9768) -> (206.2779, -294.4284)
  line L608 (206.2779, -329.9768) -> (173.8429, -329.9768)
  line L609 (173.8429, -329.9768) -> (173.8429, -316.1756)
  line L610 (173.8429, -316.1756) -> (206.2779, -316.1756)
  line L611 (206.2779, -316.1756) -> (206.2779, -329.9768)
  line L612 (206.2779, -308.973) -> (173.8429, -308.973)
  line L613 (173.8429, -308.973) -> (173.8429, -297.96)
  line L614 (173.8429, -297.96) -> (206.2779, -297.96)
  line L615 (206.2779, -297.96) -> (206.2779, -308.973)
  line L616 (242.9879, -330.0232) -> (227.2351, -330.0232)
  line L617 (227.2351, -330.0232) -> (210.553, -313.3411)
  line L618 (210.553, -313.3411) -> (210.553, -279.9768)
  line L619 (210.553, -279.9768) -> (227.2351, -279.9768)
  line L620 (227.2351, -279.9768) -> (227.2351, -315.1998)
  line L621 (227.2351, -315.1998) -> (242.9879, -315.1998)
  line L622 (242.9879, -315.1998) -> (242.9879, -330.0232)
  line L623 (246.4266, -329.9768) -> (246.4266, -279.9768)
  line L624 (246.4266, -279.9768) -> (262.8299, -279.9768)
  line L625 (262.8299, -279.9768) -> (262.8299, -313.3411)
  line L626 (262.8299, -313.3411) -> (246.4266, -329.9768)
  line L627 (283.7872, -329.9768) -> (273.4247, -329.9768)
  line L628 (273.4247, -329.9768) -> (267.105, -323.7035)
  line L629 (267.105, -323.7035) -> (267.105, -286.25)
  line L630 (267.105, -286.25) -> (273.4247, -279.9768)
  line L631 (273.4247, -279.9768) -> (299.54, -279.9768)
  line L632 (299.54, -279.9768) -> (299.54, -294.4284)
  line L633 (299.54, -294.4284) -> (283.7872, -294.4284)
  line L634 (283.7872, -294.4284) -> (283.7872, -329.9768)
  line L635 (319.6608, -323.7035) -> (313.3411, -329.9768)
  line L636 (313.3411, -329.9768) -> (287.1794, -329.9768)
  line L637 (287.1794, -329.9768) -> (287.1794, -316.1756)
  line L638 (287.1794, -316.1756) -> (302.9786, -316.1756)
  line L639 (302.9786, -316.1756) -> (302.9786, -279.9768)
  line L640 (302.9786, -279.9768) -> (313.3411, -279.9768)
  line L641 (313.3411, -279.9768) -> (319.6608, -286.25)
  line L642 (319.6608, -286.25) -> (319.6608, -323.7035)
  point P0 (0, 0)
  dimension "d71" = 150
  dimension "d72" = 50
  constraints: 2 vertical alignment, 2 other
  measures "d71" distance between parallel lines of L573 L576
  measures "d72" distance between parallel lines of L574 L576
extrude "Extrusion4" cut sketch "Sketch5" against normal blind 10 contours L578 L579 L580 L581 L582 | L583 L584 L585 L586 | L587 L588 L589 L590 L591 L592 L593 | L594 L595 L596 L597 | L598 L599 L600 L601 L602 L603 | L604 L605 L606 L607 | L608 L609 L610 L611 | L612 L613 L614 L615 | L616 L617 L618 L619 L620 L621 L622 | L623 L624 L625 L626 | L627 L628 L629 L630 L631 L632 L633 L634 | L635 L636 L637 L638 L639 L640 L641 L642
equation "\"d2\" = d0"
equation "\"d3\" = d2"
equation "\"d4\" = d3"
equation "\"d5\" = d0"
equation "\"d6\" = d0"
equation "\"d25\" = 0.5 * d11"
equation "\"d36\" = d35"
equation "\"d40\" = d39"
equation "\"d41\" = d39"
body "Solid1"
